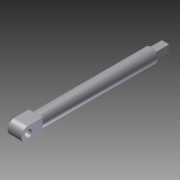
# Autodesk Inventor part: linac arm1
Saved by Autodesk Inventor 2011 (Build 150239000, 239)
## iProperties
Created: 2011-10-08
Part Number: linac arm1
Document SubType Name: Modeling
Designer: Matthew
Density: 1 g/cm^3
Author: Matthew
Autodesk Inventor part; units mm, degrees
ref_plane "YZ Plane" through (0, 0, 0) normal (1, 0, 0) x (0, 1, 0)
ref_plane "XZ Plane" through (0, 0, 0) normal (0, 1, 0) x (-1, 0, 0)
ref_plane "XY Plane" through (0, 0, 0) normal (0, 0, 1) x (1, 0, 0)
sketch "Sketch1" plane through (0, 0, 0) normal (0, 0, 1) x (1, 0, 0)
  circle A0 centre (0, 0) radius 6.0688
  constraints: 1 centre point, 1 coincident
extrude "Extrusion1" add sketch "Sketch1" along normal blind 101.6
sketch "Sketch2" plane through (0, 0, 101.6) normal (0, 0, 1) x (1, 0, 0)
  line L0 (-6.0688, 6.0688) -> (6.0688, 6.0688)
  line L1 (6.0688, 6.0688) -> (6.0688, -6.0688)
  line L2 (6.0688, -6.0688) -> (-6.0688, -6.0688)
  line L3 (-6.0688, -6.0688) -> (-6.0688, 6.0688)
  constraints: 8 end point, 2 parallel, 1 horizontal, 1 perpendicular
extrude "Extrusion2" add sketch "Sketch2" along normal blind 12.7
sketch "Sketch3" plane through (6.0688, -6.0688, 101.6) normal (1, 0, 0) x (0, 0, -1)
  line L0 (-12.7, 12.1376) -> (-12.7, 0) projected
  circle A0 centre (-12.7, 6.0688) radius 3.175
  point P0 (101.6, 6.0688)
  dimension "d4" = 6.35
  constraints: 1 centre point, 1 midpoint
  measures "d4" diameter of A0
extrude "Extrusion3" cut sketch "Sketch3" against normal blind 12.7
sketch "Sketch4" plane through (6.0688, -6.0688, 101.6) normal (1, 0, 0) x (0, 0, -1)
  arc A0 (-12.7, 2.8938) -> (-12.7, 9.2438) centre (-12.7, 6.0688) ccw projected
  circle A1 centre (-12.7, 6.0688) radius 3.175
  circle A2 centre (-12.7, 6.0688) radius 6.0688
  point P0 (101.6, 6.0688)
  constraints: 2 coincident, 1 centre point, 1 vertical alignment, 2 other
extrude "Extrusion4" add sketch "Sketch4" against normal blind 12.7
sketch "Sketch5" plane through (-6.0688, 0, 101.6) normal (-1, 0, 0) x (0, 0, 1)
  arc A0 (12.7, 6.0688) -> (12.7, -6.0688) centre (12.7, 0) ccw projected
  line L0 (0, 6.0688) -> (12.7, 6.0688) projected
  line L1 (0, 0) -> (0, 6.0688) projected
  line L2 (0, -6.0688) -> (0, 0) projected
  line L3 (0, -6.0688) -> (12.7, -6.0688) projected
  line L4 (0, 6.0688) -> (38.3978, 6.0688)
  line L5 (38.3978, 6.0688) -> (38.3978, -6.0688)
  line L6 (38.3978, -6.0688) -> (0, -6.0688)
  line L7 (0, -6.0688) -> (0, 6.0688)
  point P0 (-101.6, 0)
  constraints: 8 end point, 2 parallel, 1 horizontal, 1 perpendicular
extrude "Extrusion5" cut sketch "Sketch5" along normal blind 12.7 contours L4 L5 L6 A0
sketch "Sketch6" plane through (0, 0, 0) normal (0, 0, -1) x (-1, 0, 0)
  circle A0 centre (0, 0) radius 6.0688 projected
  line L0 (0, 0) -> (0, 3.175)
  line L1 (0, 3.175) -> (-3.175, 3.175)
  line L2 (-3.175, 3.175) -> (3.175, 3.175)
  line L3 (3.175, 3.175) -> (3.175, -3.175)
  line L4 (3.175, -3.175) -> (-3.175, -3.175)
  line L5 (-3.175, -3.175) -> (-3.175, 3.175)
  dimension "d11" = 3.175
  dimension "d12" = 3.175
  dimension "d13" = 6.35
  dimension "d14" = 6.35
  constraints: 12 end point, 2 parallel, 2 perpendicular, 1 horizontal, 1 vertical
  measures "d11" distance of L0.start L0.end
  measures "d12" distance of L0.end L1.end
  measures "d13" distance of L3.end L4.end
  measures "d14" distance of L2.end L3.end
extrude "Extrusion6" add sketch "Sketch6" along normal blind 12.7 contours L2 L3 L4 L5 L1
body "Solid1"
